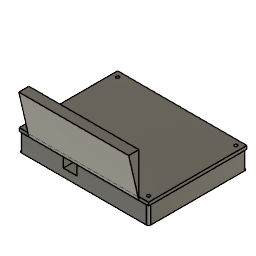
inky_case (Autodesk Fusion 360 design; units mm, degrees)
Autodesk Fusion 360 part; units mm, degrees
sketch "Sketch1" plane through (0, 0, 0) normal (0, 0, 1) x (1, 0, 0)
  line L0 (-58.8, -44.75) -> (58.8, -44.75)
  line L1 (58.8, -44.75) -> (58.8, 44.75)
  line L2 (58.8, 44.75) -> (-58.8, 44.75)
  line L3 (-58.8, 44.75) -> (-58.8, -44.75)
extrude "Extrude1" add sketch "Sketch1" along normal blind 16 makes body 1
ref_plane "WorkPlane1" through (0, 0, 2) normal (0, 0, 1) x (1, 0, 0)
sketch "Sketch2" plane through (0, 0, 2) normal (0, 0, 1) x (1, 0, 0)
  line L0 (-48.8, -34.75) -> (48.8, -34.75)
  line L1 (48.8, -34.75) -> (48.8, 34.75)
  line L2 (48.8, 34.75) -> (-48.8, 34.75)
  line L3 (-48.8, 34.75) -> (-48.8, -34.75)
extrude "Extrude2" add sketch "Sketch2" along normal blind 15 separate body makes body 2
combine "Combine1" operation cut target body 1 tool bodies 2
ref_plane "WorkPlane2" through (0, 0, -1) normal (0, 0, 1) x (1, 0, 0)
sketch "Sketch3" plane through (0, 0, -1) normal (0, 0, 1) x (1, 0, 0)
  line L0 (-43, -25.85) -> (43, -25.85)
  line L1 (43, -25.85) -> (43, 28.15)
  line L2 (43, 28.15) -> (-43, 28.15)
  line L3 (-43, 28.15) -> (-43, -25.85)
extrude "Extrude3" add sketch "Sketch3" along normal blind 4 separate body makes body 3
combine "Combine2" operation cut target body 1 tool bodies 3
ref_plane "WorkPlane3" through (0, -45.25, 0) normal (0, 1, 0) x (0, 0, 1)
sketch "Sketch4" plane through (0, -45.25, 0) normal (0, 1, 0) x (1, 0, 0)
  line L0 (-18.7, -7.2) -> (-6.3, -7.2)
  line L1 (-6.3, -7.2) -> (-6.3, -17.8)
  line L2 (-6.3, -17.8) -> (-18.7, -17.8)
  line L3 (-18.7, -17.8) -> (-18.7, -7.2)
extrude "Extrude4" add sketch "Sketch4" along normal blind 11 separate body makes body 4
combine "Combine3" operation cut target body 1 tool bodies 4
ref_plane "WorkPlane4" through (0, 0, 11) normal (0, 0, 1) x (1, 0, 0)
sketch "Sketch5" plane through (0, 0, 11) normal (0, 0, 1) x (1, 0, 0)
  circle A0 centre (-53.8, -39.75) radius 1
extrude "Extrude5" add sketch "Sketch5" along normal blind 5 separate body makes body 5
combine "Combine4" operation cut target body 1 tool bodies 5
ref_plane "WorkPlane5" through (0, 0, 11) normal (0, 0, 1) x (1, 0, 0)
sketch "Sketch6" plane through (0, 0, 11) normal (0, 0, 1) x (1, 0, 0)
  circle A0 centre (-53.8, 39.75) radius 1
extrude "Extrude6" add sketch "Sketch6" along normal blind 5 separate body makes body 6
combine "Combine5" operation cut target body 1 tool bodies 6
ref_plane "WorkPlane6" through (0, 0, 11) normal (0, 0, 1) x (1, 0, 0)
sketch "Sketch7" plane through (0, 0, 11) normal (0, 0, 1) x (1, 0, 0)
  circle A0 centre (53.8, -39.75) radius 1
extrude "Extrude7" add sketch "Sketch7" along normal blind 5 separate body makes body 7
combine "Combine6" operation cut target body 1 tool bodies 7
ref_plane "WorkPlane7" through (0, 0, 11) normal (0, 0, 1) x (1, 0, 0)
sketch "Sketch8" plane through (0, 0, 11) normal (0, 0, 1) x (1, 0, 0)
  circle A0 centre (53.8, 39.75) radius 1
extrude "Extrude8" add sketch "Sketch8" along normal blind 5 separate body makes body 8
combine "Combine7" operation cut target body 1 tool bodies 8
fillet "Fillet1" radius 2 4 edges at (-58.8, -44.75, 8) (58.8, -44.75, 8) (-58.8, 44.75, 8) (58.8, 44.75, 8) on bodies 1
ref_plane "WorkPlane8" through (0, 0, 16) normal (0, 0, 1) x (1, 0, 0)
sketch "Sketch9" plane through (0, 0, 16) normal (0, 0, 1) x (1, 0, 0)
  line L0 (-58.8, -44.75) -> (58.8, -44.75)
  line L1 (58.8, -44.75) -> (58.8, 44.75)
  line L2 (58.8, 44.75) -> (-58.8, 44.75)
  line L3 (-58.8, 44.75) -> (-58.8, -44.75)
extrude "Extrude9" add sketch "Sketch9" along normal blind 3 separate body makes body 9
ref_plane "WorkPlane9" through (-50, 0, 0) normal (1, 0, 0) x (0, 1, 0)
sketch "Sketch10" plane through (-50, 0, 0) normal (1, 0, 0) x (0, 0, -1)
  line L0 (-16, -44.75) -> (-56, -44.75)
  line L1 (-56, -44.75) -> (-56, -53.9847)
  line L2 (-56, -53.9847) -> (-16, -44.75)
extrude "Extrude10" add sketch "Sketch10" along normal blind 100 separate body makes body 10
combine "Combine8" operation add target body 9 tool bodies 10
ref_plane "WorkPlane10" through (0, 0, 15) normal (0, 0, 1) x (1, 0, 0)
sketch "Sketch11" plane through (0, 0, 15) normal (0, 0, 1) x (1, 0, 0)
  circle A0 centre (-53.8, -39.75) radius 1.4
extrude "Extrude11" add sketch "Sketch11" along normal blind 5 separate body makes body 11
combine "Combine9" operation cut target body 9 tool bodies 11
ref_plane "WorkPlane11" through (0, 0, 15) normal (0, 0, 1) x (1, 0, 0)
sketch "Sketch12" plane through (0, 0, 15) normal (0, 0, 1) x (1, 0, 0)
  circle A0 centre (-53.8, 39.75) radius 1.4
extrude "Extrude12" add sketch "Sketch12" along normal blind 5 separate body makes body 12
combine "Combine10" operation cut target body 9 tool bodies 12
ref_plane "WorkPlane12" through (0, 0, 15) normal (0, 0, 1) x (1, 0, 0)
sketch "Sketch13" plane through (0, 0, 15) normal (0, 0, 1) x (1, 0, 0)
  circle A0 centre (53.8, -39.75) radius 1.4
extrude "Extrude13" add sketch "Sketch13" along normal blind 5 separate body makes body 13
combine "Combine11" operation cut target body 9 tool bodies 13
ref_plane "WorkPlane13" through (0, 0, 15) normal (0, 0, 1) x (1, 0, 0)
sketch "Sketch14" plane through (0, 0, 15) normal (0, 0, 1) x (1, 0, 0)
  circle A0 centre (53.8, 39.75) radius 1.4
extrude "Extrude14" add sketch "Sketch14" along normal blind 5 separate body makes body 14
combine "Combine12" operation cut target body 9 tool bodies 14
ref_plane "WorkPlane14" through (0, 0, 4.5) normal (0, 0, 1) x (1, 0, 0)
sketch "Sketch15" plane through (0, 0, 4.5) normal (0, 0, 1) x (1, 0, 0)
  circle A0 centre (-44.4, -30.35) radius 3
extrude "Extrude15" add sketch "Sketch15" along normal blind 11.5 separate body makes body 15
combine "Combine13" operation add target body 9 tool bodies 15
ref_plane "WorkPlane15" through (0, 0, 4.5) normal (0, 0, 1) x (1, 0, 0)
sketch "Sketch16" plane through (0, 0, 4.5) normal (0, 0, 1) x (1, 0, 0)
  circle A0 centre (-44.4, 30.35) radius 3
extrude "Extrude16" add sketch "Sketch16" along normal blind 11.5 separate body makes body 16
combine "Combine14" operation add target body 9 tool bodies 16
ref_plane "WorkPlane16" through (0, 0, 4.5) normal (0, 0, 1) x (1, 0, 0)
sketch "Sketch17" plane through (0, 0, 4.5) normal (0, 0, 1) x (1, 0, 0)
  circle A0 centre (44.4, -30.35) radius 3
extrude "Extrude17" add sketch "Sketch17" along normal blind 11.5 separate body makes body 17
combine "Combine15" operation add target body 9 tool bodies 17
ref_plane "WorkPlane17" through (0, 0, 4.5) normal (0, 0, 1) x (1, 0, 0)
sketch "Sketch18" plane through (0, 0, 4.5) normal (0, 0, 1) x (1, 0, 0)
  circle A0 centre (44.4, 30.35) radius 3
extrude "Extrude18" add sketch "Sketch18" along normal blind 11.5 separate body makes body 18
combine "Combine16" operation add target body 9 tool bodies 18
